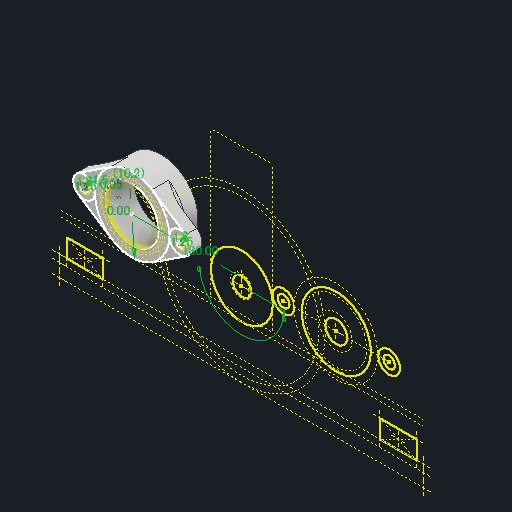
# Autodesk Inventor part: encodersupporter
Saved by Autodesk Inventor 2023.5 (Build 275446000, 446)
## iProperties
Created: 2025-01-19
Part Number: encodersupporter
Material: 一般
Document SubType Name: Modeling
Designer: IshiiLabHonda
Density: 1 g/cm^3
Appearance: 既定
Author: IshiiLabHonda
Autodesk Inventor part; units mm, degrees
ref_plane "YZ Plane" through (0, 0, 0) normal (1, 0, 0) x (0, 1, 0)
ref_plane "XZ Plane" through (0, 0, 0) normal (0, 1, 0) x (-1, 0, 0)
ref_plane "XY Plane" through (0, 0, 0) normal (0, 0, 1) x (1, 0, 0)
derived "motormount-l.ipt"
sketch "スケッチ1" plane through (0, 0, 0) normal (0, 0, 1) x (1, 0, 0)
  circle A0 centre (0, 0) radius 10.65 construction
  line L0 (0, 0) -> (0, 1) construction
  line L1 (0, 0) -> (1, 0) construction
  circle A1 centre (12.953378, 1.1) radius 2.25 construction
  circle A2 centre (-15.066851, 1) radius 4.35 construction
  circle A3 centre (0, 0) radius 11.5 construction
  line L2 (-25, -11.5) -> (25, -11.5) construction
  line L3 (-25, -9.7) -> (25, -9.7) construction
  line L4 (-25, -8.7) -> (25, -8.7) construction
  line L5 (-25, -4.2) -> (25, -4.2) construction
  line L6 (-25, -3.4) -> (25, -3.4) construction
  line L7 (-4.25, 16.6) -> (-4.25, -3.4) construction
  line L8 (4.25, 16.6) -> (4.25, -3.4) construction
  line L9 (-4.25, 16.6) -> (4.25, 16.6) construction
sketch "スケッチ2" plane through (0, 0, 0) normal (0, 0, 1) x (1, 0, 0)
  circle A0 centre (-15.066851, 1) radius 4.35 construction
  line L0 (0, 0) -> (0, 1) construction
  circle A1 centre (0, 0) radius 10.65 construction
  circle A2 centre (0, 0) radius 11.5 construction
  line L1 (-25, -8.7) -> (25, -8.7) construction
  line L2 (-25, -9.7) -> (25, -9.7) construction
  line L3 (-25, -11.5) -> (25, -11.5) construction
  line L4 (0, 0) -> (1, 0) construction
  circle A3 centre (12.953378, 1.1) radius 2.25 construction
  circle A4 centre (12.953378, 1.1) radius 4.25 construction
  circle A5 centre (-15.066851, 1) radius 3.6 construction
  circle A6 centre (-15.066851, 1) radius 3 construction
  circle A7 centre (0, 0) radius 1.25 construction
  circle A8 centre (0, 0) radius 1.5 construction
sketch "スケッチ3" plane through (0, 0, 0) normal (0, 0, 1) x (1, 0, 0)
  circle A0 centre (-15.066851, 1) radius 4.35 construction
  line L0 (0, 0) -> (0, 1) construction
  line L1 (0, 0) -> (1, 0) construction
  line L2 (-25, -11.5) -> (25, -11.5) construction
  line L3 (-25, -9.7) -> (25, -9.7) construction
  line L4 (-25, -8.7) -> (25, -8.7) construction
  circle A1 centre (12.953378, 1.1) radius 2.25 construction
  circle A2 centre (0, 0) radius 10.65 construction
  circle A3 centre (0, 0) radius 11.5 construction
  circle A4 centre (-15.066851, 1) radius 4.35 construction
  line L5 (0, 0) -> (0, 1) construction
  circle A5 centre (0, 0) radius 10.65 construction
  circle A6 centre (0, 0) radius 11.5 construction
  line L6 (-25, -8.7) -> (25, -8.7) construction
  line L7 (-25, -9.7) -> (25, -9.7) construction
  line L8 (-25, -11.5) -> (25, -11.5) construction
  line L9 (0, 0) -> (1, 0) construction
  circle A7 centre (12.953378, 1.1) radius 2.25 construction
  circle A8 centre (12.953378, 1.1) radius 4.25 construction
  circle A9 centre (-15.066851, 1) radius 3.6 construction
  circle A10 centre (-15.066851, 1) radius 3 construction
  line L10 (-24, -6.2) -> (-19, -6.2)
  line L11 (-19, -6.2) -> (-19, -8.7)
  line L12 (-24, -8.7) -> (-24, -6.2)
  line L13 (19, -6.2) -> (24, -6.2)
  line L14 (24, -6.2) -> (24, -8.7)
  line L15 (19, -8.7) -> (19, -6.2)
  line L16 (-24, -6.2) -> (-19, -8.7) construction
  line L17 (-24, -8.7) -> (-19, -6.2) construction
  line L18 (19, -6.2) -> (24, -8.7) construction
  line L19 (19, -8.7) -> (24, -6.2) construction
  line L20 (-24, -8.7) -> (-19, -8.7)
  line L21 (19, -8.7) -> (24, -8.7)
  circle A11 centre (-15.066851, 1) radius 3.2 construction
  circle A12 centre (-15.066851, 1) radius 4.1 construction
  circle A13 centre (12.953378, 1.1) radius 4.75
  circle A14 centre (0, 0) radius 4.25
  circle A15 centre (0, 0) radius 1.25
  circle A16 centre (12.953378, 1.1) radius 1.5
  line L22 (-4.25, 16.6) -> (-4.25, -3.4) construction
  line L23 (-4.25, 16.6) -> (4.25, 16.6) construction
  line L24 (4.25, 16.6) -> (4.25, -3.4) construction
  line L25 (-25, -3.4) -> (25, -3.4) construction
  line L26 (-25, -4.2) -> (25, -4.2) construction
  circle A17 centre (12.953378, 1.1) radius 5.75 construction
  circle A18 centre (20.203378, 1.1) radius 1.5
  circle A19 centre (20.203378, 1.1) radius 0.8
  circle A20 centre (5.703378, 1.1) radius 0.8
  circle A21 centre (5.703378, 1.1) radius 1.5
  line L27 (5.703378, 1.1) -> (12.953378, 1.1) construction
  line L28 (12.953378, 1.1) -> (20.203378, 1.1) construction
  circle A22 centre (-15.066851, 1) radius 5.1 construction
  circle A23 centre (-21.666851, 1) radius 0.8
  circle A24 centre (-21.666851, 1) radius 1.5
  circle A25 centre (-8.466851, 1) radius 0.8
  circle A26 centre (-8.466851, 1) radius 1.5
  line L29 (-21.666851, 1) -> (-15.066851, 1) construction
  line L30 (-15.066851, 1) -> (-8.466851, 1) construction
  point P0 (-21.5, -7.45)
  point P1 (21.5, -7.45)
sketch "スケッチ4" plane through (0, 0, 0) normal (0, 0, 1) x (1, 0, 0)
  circle A0 centre (-21.666851, 1) radius 1.5
  circle A1 centre (-21.666851, 1) radius 0.625
  circle A2 centre (-21.666851, 1) radius 0.8 construction
  circle A3 centre (0, 0) radius 10.65 construction
  line L0 (0, 0) -> (0, 1) construction
  line L1 (0, 0) -> (1, 0) construction
  circle A4 centre (12.953378, 1.1) radius 2.25 construction
  circle A5 centre (-15.066851, 1) radius 4.35 construction
  circle A6 centre (0, 0) radius 11.5 construction
  line L2 (-25, -11.5) -> (25, -11.5) construction
  line L3 (-25, -9.7) -> (25, -9.7) construction
  line L4 (-25, -8.7) -> (25, -8.7) construction
  circle A7 centre (-15.066851, 1) radius 4.35 construction
  line L5 (0, 0) -> (0, 1) construction
  circle A8 centre (0, 0) radius 10.65 construction
  circle A9 centre (0, 0) radius 11.5 construction
  line L6 (-25, -8.7) -> (25, -8.7) construction
  line L7 (-25, -9.7) -> (25, -9.7) construction
  line L8 (-25, -11.5) -> (25, -11.5) construction
  line L9 (0, 0) -> (1, 0) construction
  circle A10 centre (12.953378, 1.1) radius 2.25 construction
  circle A11 centre (12.953378, 1.1) radius 4.25 construction
  circle A12 centre (-15.066851, 1) radius 3.6 construction
  circle A13 centre (-15.066851, 1) radius 3 construction
  circle A14 centre (0, 0) radius 1.25 construction
  circle A15 centre (0, 0) radius 1.5 construction
  line L10 (-25, -11.5) -> (25, -11.5) construction
  line L11 (-25, -11.5) -> (25, -11.5) construction
  line L12 (-25, -9.7) -> (25, -9.7) construction
  line L13 (-25, -9.7) -> (25, -9.7) construction
  line L14 (-25, -8.7) -> (25, -8.7) construction
  line L15 (0, 0) -> (1, 0) construction
  line L16 (0, 0) -> (1, 0) construction
  line L17 (0, 0) -> (0, 1) construction
  line L18 (0, 0) -> (0, 1) construction
  circle A16 centre (0, 0) radius 1.25
  circle A17 centre (12.953378, 1.1) radius 2.25 construction
  circle A18 centre (0, 0) radius 4.25
  circle A19 centre (0, 0) radius 11.5 construction
  circle A20 centre (0, 0) radius 11.5 construction
  circle A21 centre (0, 0) radius 10.65 construction
  circle A22 centre (0, 0) radius 10.65 construction
  circle A23 centre (-15.066851, 1) radius 4.35 construction
  circle A24 centre (-15.066851, 1) radius 4.35 construction
  line L19 (-25, -8.7) -> (25, -8.7) construction
  circle A25 centre (-15.066851, 1) radius 3 construction
  circle A26 centre (-15.066851, 1) radius 3.2 construction
  circle A27 centre (-15.066851, 1) radius 3.6
  circle A28 centre (-15.066851, 1) radius 4.1 construction
  circle A29 centre (12.953378, 1.1) radius 1.5
  circle A30 centre (12.953378, 1.1) radius 2.25 construction
  circle A31 centre (12.953378, 1.1) radius 4.25 construction
  circle A32 centre (12.953378, 1.1) radius 4.75
  line L20 (19, -8.7) -> (19, -6.2)
  line L21 (19, -6.2) -> (24, -6.2)
  line L22 (19, -8.7) -> (24, -8.7)
  line L23 (19, -6.2) -> (24, -8.7) construction
  line L24 (24, -6.2) -> (24, -8.7)
  line L25 (19, -8.7) -> (24, -6.2) construction
  line L26 (-19, -6.2) -> (-19, -8.7)
  line L27 (-24, -8.7) -> (-24, -6.2)
  line L28 (-24, -6.2) -> (-19, -8.7) construction
  line L29 (-24, -8.7) -> (-19, -6.2) construction
  line L30 (-24, -8.7) -> (-19, -8.7)
  line L31 (-24, -6.2) -> (-19, -6.2)
  circle A33 centre (-15.066851, 1) radius 3.65
  circle A34 centre (-15.066851, 1) radius 5.1
  circle A35 centre (-8.466851, 1) radius 1.5
  circle A36 centre (-8.466851, 1) radius 0.625
  circle A37 centre (-8.466851, 1) radius 0.8 construction
  line L32 (-15.066851, 1) -> (-21.666851, 1) construction
  line L33 (-15.066851, 1) -> (-8.466851, 1) construction
  line L34 (-22.485033, 2.257211) -> (-17.848669, 5.274516)
  line L35 (-12.285033, 5.274516) -> (-7.648669, 2.257211)
  line L36 (-7.648669, -0.257211) -> (-12.285033, -3.274516)
  line L37 (-17.848669, -3.274516) -> (-22.485033, -0.257211)
  point P0 (21.5, -7.45)
  point P1 (-21.5, -7.45)
  point P2 (-9.966851, 1)
  point P3 (-20.166851, 1)
  dimension "d1" = 1.25
  dimension "d2" = 1.6
  dimension "d3" = 3
  dimension "d4" = 0.05
  dimension "d5" = 1.5
  dimension "d6" = 1.25
  dimension "d7" = 1.6
  dimension "d8" = 3
  dimension "d13" = 0
  dimension "d14" = 0
  dimension "d15" = 10.2
  constraints: 12 end point, 10 tangent, 8 centre point, 8 point on circle, 6 coincident, 9 other
  measures "d1" diameter of A1
  measures "d2" diameter of A2
  measures "d3" diameter of A0
  measures "d4" radial gap between concentric circles of A12 A33
  measures "d5" radial gap between concentric circles of A34 A12
  measures "d6" diameter of A36
  measures "d7" diameter of A37
  measures "d8" diameter of A35
  measures "d13" vertical extent of L33
  measures "d14" vertical extent of L32
  measures "d15" diameter of A34
extrude "押し出し1" add sketch "スケッチ4" against normal blind 4 contours A34
extrude "押し出し2" add sketch "スケッチ4" against normal blind 1.5 contours A0 | A35
extrude "押し出し3" add sketch "スケッチ4" against normal blind 1.5 contours A34 L37 A0 | A0 L34 A34 | L35 A35 A34 | A34 A35 L36
fillet "フィレット1" radius 0.8 3 edges at (-10.5837, 3.4313, -1.5) (-10.5837, -1.4313, -1.5) (-20.1669, 1, -1.5)
